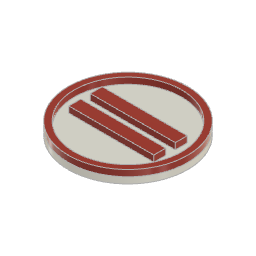
_Straight.5817e1ad-5611-4c21-aade-69f26989d87a (Autodesk Fusion 360 design; units mm, degrees)
Autodesk Fusion 360 part; units mm, degrees
sketch "Sketch1" plane through (0, 0, 0) normal (0, 0, 1) x (1, 0, 0)
  circle A0 centre (0, 0) radius 15.875
  circle A1 centre (0, 0) radius 14.2875
  line L0 (0, 0) -> (14.2875, 0)
  line L1 (0, 0) -> (5.6434, 0)
  line L2 (5.6434, 1.27) -> (0, 1.27)
  line L3 (0, 1.27) -> (11.3127, 1.27)
  line L4 (11.3127, 1.27) -> (11.3127, 4.445)
  line L5 (11.3127, 4.445) -> (0, 4.445)
  line L6 (-5.6434, 1.27) -> (0, 1.27)
  line L7 (0, 1.27) -> (-11.3127, 1.27)
  line L8 (-11.3127, 4.445) -> (0, 4.445)
  line L9 (-11.3127, 1.27) -> (-11.3127, 4.445)
  line L10 (-11.3127, 4.445) -> (11.3127, 4.445)
  line L11 (11.3127, 4.445) -> (11.3127, 1.27)
  line L12 (11.3127, 1.27) -> (-11.3127, 1.27)
  line L13 (-11.3127, 1.27) -> (-11.3127, 4.445)
  line L14 (5.6434, -1.27) -> (0, -1.27)
  line L15 (-11.3127, -1.27) -> (-11.3127, -4.445)
  line L16 (-5.6434, -1.27) -> (0, -1.27)
  line L17 (11.3127, -4.445) -> (11.3127, -1.27)
  line L18 (11.3127, -4.445) -> (0, -4.445)
  line L19 (-11.3127, -4.445) -> (0, -4.445)
  line L20 (-11.3127, -1.27) -> (-11.3127, -4.445)
  line L21 (0, -1.27) -> (11.3127, -1.27)
  line L22 (0, -1.27) -> (-11.3127, -1.27)
  line L23 (-11.3127, -4.445) -> (11.3127, -4.445)
  line L24 (11.3127, -1.27) -> (11.3127, -4.445)
  line L25 (11.3127, -1.27) -> (-11.3127, -1.27)
  dimension "d17" = 1.27
  dimension "d18" = 3.175
  constraint coincident A0.centre A1.centre
  constraint coincident A1 L0.end
  constraint horizontal L0
  constraint horizontal L1
  constraint horizontal L2
  constraint horizontal L3
  constraint vertical L4
  constraint horizontal L5
  constraint horizontal L10
  constraint vertical L11
  constraint horizontal L12
  constraint vertical L13
  constraint symmetric L0 L2.start L14.start
  constraint symmetric L0 L2.end L14.end
  constraint symmetric L0 L3.end L17.end
  constraint symmetric L0 L4.end L17.start
  constraint symmetric L0 L5.end L18.end
  constraint symmetric L0 L7.end L15.start
  constraint symmetric L0 L8.start L15.end
  constraint symmetric L0 L6.start L16.start
  measures "d17" distance of A0.centre L2.end
  measures "d18" distance of L2.end L5.end
extrude "Extrude1" add sketch "Sketch1" against normal blind 1 contours A0 | A1 | L2 L3 L4 L5 L6 L7 L8 L9 L10 L11 L12 L13 | L14 L15 L16 L17 L18 L19 L20 L21 L22 L23 L24 L25 makes body 1 in component "Base"
extrude "Extrude1'" add sketch "Sketch1" along normal blind 1 separate body makes body 2 at (15.2335, -1.4985, 0) makes body 3 at (-3.7709, -3.3867, 0) makes body 4 at (-3.7709, 2.3283, 0) in component "Top"
scale "Scale1" factors (0.6, 0.6, 1) about (-11.3127, -4.445, 0) bodies 3 2 4 in component "Top"
scale "Scale1'" factors (0.6, 0.6, 1) about (-11.3127, -4.445, 0) bodies 1 in component "Base"
component "Base" placed x (1, 0, 0) y (0, 1, 0) z (0, 0, 1) at (0, 0, 0)
component "Top" placed x (1, 0, 0) y (0, 1, 0) z (0, 0, 1) at (0, 0, 0)
